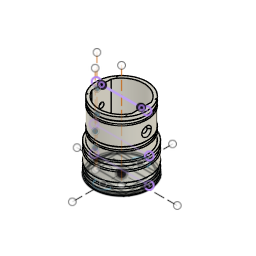
Gehäuse_unten v17 (Autodesk Fusion 360 design; units mm, degrees)
Autodesk Fusion 360 part; units mm, degrees
note: some values were not read from the file. Set by a fixed rule: which sketch regions a step uses; the direction of a hole.
sketch "Skizze1" plane through (0, 0, 0) normal (0, 0, 1) x (1, 0, 0)
  circle A0 centre (0, 0) radius 24.75
  circle A1 centre (0, 0) radius 21.75
  line L0 (-17.5, 13.5) -> (17.5, 13.5)
  line L1 (17.5, 13.5) -> (17.5, -13.5)
  line L2 (17.5, -13.5) -> (-17.5, -13.5)
  line L3 (-17.5, -13.5) -> (-17.5, 13.5)
  line L4 (-40, 0) -> (50, 0) construction
  line L5 (0, 45.7661) -> (0, -44.2339) construction
  line L6 (-18.4476, 16.5) -> (18.4476, 16.5)
  line L7 (20.5, 13.8677) -> (20.5, -13.8677)
  line L8 (18.4476, -16.5) -> (-18.4476, -16.5)
  line L9 (-20.5, -13.8677) -> (-20.5, 13.8677)
  arc A2 (6.5, 16.5) -> (-6.5, 16.5) centre (0, 16.5) ccw
  arc A3 (-6.6213, -16.5) -> (6.3787, -16.5) centre (-0.1213, -16.5) ccw
  arc A4 (-21.6357, 2.2272) -> (-21.6357, -2.2272) centre (-20.5, 0) ccw
  arc A5 (20.5, -2.5) -> (20.5, 2.5) centre (20.5, 0) ccw
  circle A6 centre (0, 0) radius 23 construction
  line L10 (-14.5, -7.5) -> (14.5, -7.5)
  line L11 (14.5, -7.5) -> (14.5, 7.5)
  line L12 (14.5, 7.5) -> (-14.5, 7.5)
  line L13 (-14.5, 7.5) -> (-14.5, -7.5)
  circle A7 centre (0, 0) radius 22.75
  dimension "d1" = 49.5
  dimension "d3" = 3
  dimension "d4" = 27
  dimension "d5" = 35
  dimension "d6" = 3
  dimension "d7" = 3
  dimension "d8" = 3
  dimension "d9" = 3
  dimension "d18" = 46
  dimension "d19" = 29
  dimension "d20" = 15
  dimension "d43" = 45.5
  constraint coincident A0.centre A1.centre
  constraint horizontal L0
  constraint vertical L1
  constraint horizontal L2
  constraint vertical L3
  constraint parallel L2 L4
  constraint symmetric L0 L2 L4
  constraint vertical L5
  constraint symmetric L1 L3 L5
  constraint coincident A0.centre L5
  constraint coincident A0.centre L4
  constraint horizontal L6
  constraint vertical L7
  constraint horizontal L8
  constraint vertical L9
  constraint equal A2 A3
  constraint coincident L6 A2.end
  constraint coincident L6 A2.start
  constraint coincident L8 A3.end
  constraint coincident L8 A3.start
  constraint coincident A0 L8.end
  constraint coincident L8 A3.centre
  constraint coincident A0 L9.start
  constraint coincident A0 L9.end
  constraint coincident A0 L6.start
  constraint coincident L6 A2.centre
  constraint coincident A0 L7.start
  constraint coincident A0 L6.end
  constraint coincident A0 L7.end
  constraint coincident A0 L8.start
  constraint midpoint L9 A4.centre
  constraint midpoint L7 A5.centre
  constraint equal A4 A5
  constraint coincident A1 A4.start
  constraint coincident A1 A4.end
  constraint coincident L7 A5.end
  constraint coincident L7 A5.start
  constraint concentric A0 A6
  constraint tangent A5 A6
  constraint tangent A2 A6
  constraint horizontal L10
  constraint vertical L11
  constraint horizontal L12
  constraint vertical L13
  constraint symmetric L5 L11 L13
  constraint symmetric L4 L10 L12
  constraint concentric A1 A7
  measures "d1" diameter of A0
  measures "d3" distance of A0 A1
  measures "d4" distance of L0.start L2.end
  measures "d5" distance of L0.start L0.end
  measures "d6" distance of L3 L9
  measures "d7" distance of L1 L7
  measures "d8" distance of L0 L6
  measures "d9" distance of L2 L8
  measures "d18" diameter of A6
  measures "d19" distance of L10.start L10.end
  measures "d20" distance of L10.end L11.end
  measures "d43" diameter of A7
extrude "Extrusion1" add sketch "Skizze1" along normal blind 60 contours A0 L7 A5 A7 | A0 L6 L7 A7 | A0 L7 L8 A7 | A0 L6 A2 A7 | A1 L7 A5 A7 | A1 L0 L1 L6 L7 A7 | A0 L8 A3 A7 | A1 L1 L2 L7 L8 A7 | A1 L7 A5 A7 | A0 L6 L9 A7 | A1 L6 A2 A7 | A1 A5 A7 | A5 A7 | A0 L8 L9 A7 | A1 L8 A3 A7 | A0 L9 A4 A7 | A1 L6 A2 A7 | A1 L0 L3 L6 L9 A7 | A2 A7 | A1 A2 A7 | A1 L2 L3 L8 L9 A7 | A1 L8 A3 A7 | A1 A3 A7 | A3 A7 | A1 L9 A4 A7 | A1 L9 A4 A7 | A4 A7 | A1 A4 A7
extrude "Extrusion2" add sketch "Skizze1" along normal blind 3 contours A1 L1 L7 | A1 L7 A5 | A1 L7 A5 | A1 L6 A2 | A1 L0 L6 | A1 L7 A5 | A1 L0 L1 L2 L3 | A1 L2 L8 | A1 L8 A3 | A1 L6 A2 | A1 L6 A2 | A1 L8 A3 | A1 L8 A3 | A1 L9 | A1 L3 L9 | L10 L11 L12 L13
chamfer "Fase1" distance 3 angle 12 1 edges at (-23.0751, -8.95, 0) measured on face at (24.627, -2.4643, 20)
extrude "Extrusion3" cut sketch "Skizze1" along normal up to surface (3 mm away) contours L10 L11 L12 L13
extrude "Extrusion4" add sketch "Skizze1" along normal up to surface (60 mm away) contours A1 L7 A5 | A1 L7 A5 | A1 L7 A5 | A1 L9
chamfer "Fase2" distance 1.5 angle 45 4 edges at (0, -7.5, 3) (-14.5, 0, 3) (0, 7.5, 3) (14.5, 0, 3) measured on face at (-0.5022, -12.2326, 3) measured on face at (-0.5022, -12.2326, 3) measured on face at (-0.5022, -12.2326, 3) measured on face at (-0.5022, -12.2326, 3)
sketch "Skizze2" plane through (-20.5, 0, 0) normal (1, 0, 0) x (0, 1, 0)
  line L0 (-7.2672, 3) -> (7.2672, 3)
  line L1 (7.2672, 3) -> (7.2672, 60)
  line L2 (7.2672, 60) -> (-7.2672, 60)
  line L3 (-7.2672, 60) -> (-7.2672, 3)
  line L4 (7.2672, 3) -> (12.9156, 3)
  line L5 (13.5, 3) -> (12.9156, 3)
  line L6 (13.5, 3) -> (21.75, 3)
  line L7 (13.5, 3) -> (12.9156, 3)
  line L8 (7.2672, 3) -> (12.9156, 3)
  line L9 (7.2672, 3) -> (-7.2672, 3)
  line L10 (-12.9156, 3) -> (-7.2672, 3)
  line L11 (-12.9156, 3) -> (-13.5, 3)
  line L12 (-21.75, 3) -> (-13.5, 3)
  line L13 (-12.9156, 3) -> (-13.5, 3)
  line L14 (-12.9156, 3) -> (-7.2672, 3)
  line L15 (-7.2672, 3) -> (7.2672, 3)
  line L16 (-9, 3) -> (9, 3)
  line L17 (9, 3) -> (-9, 3)
  line L18 (-21.75, 60) -> (-13.5, 60)
  line L19 (-13.5, 60) -> (-12.9156, 60)
  line L20 (-12.9156, 60) -> (-7.2672, 60)
  line L21 (-7.2672, 60) -> (7.2672, 60)
  line L22 (7.2672, 60) -> (12.9156, 60)
  line L23 (12.9156, 60) -> (13.5, 60)
  line L24 (13.5, 60) -> (21.75, 60)
  line L25 (13.5, 60) -> (12.9156, 60)
  line L26 (7.2672, 60) -> (12.9156, 60)
  line L27 (7.2672, 60) -> (-7.2672, 60)
  line L28 (-12.9156, 60) -> (-7.2672, 60)
  line L29 (-12.9156, 60) -> (-13.5, 60)
  line L30 (24.75, 60) -> (-24.75, 60)
  circle A0 centre (0, 44) radius 2.25
  line L31 (0, 60) -> (0, 3) construction
  dimension "d30" = 4.5
  dimension "d31" = 41
  constraint midpoint L21 L31.start
  constraint coincident A0.centre L31
  measures "d30" diameter of A0
  measures "d31" distance of L0 A0.centre
extrude "Extrusion5" cut sketch "Skizze2" along normal blind 110 and the other way blind 40 contours A0
hole "Bohrung1" at (-0.1213, -16.5, 0) at (20.5, 0, 0) at (0, 16.5, 0) at (-20.5, 0, 0) direction (0, 0, 1) diameter 2 depth 8 tip angle 118
sketch "Skizze4" plane through (0, 0, 3) normal (0, 0, 1) x (-1, 0, 0)
  arc A0 (-20.5, -1) -> (-20.5, 1) centre (-20.5, 0) ccw
  line L0 (-20.5, -1) -> (-20.5, -7.2672)
  arc A1 (-20.5, -7.2672) -> (-17.5, -12.9156) centre (0, 0) ccw
  arc A2 (-17.5, -12.9156) -> (-17.0532, -13.5) centre (0, 0) ccw
  arc A3 (-17.0532, -13.5) -> (17.0532, -13.5) centre (0, 0) ccw
  arc A4 (17.0532, -13.5) -> (17.5, -12.9156) centre (0, 0) ccw
  arc A5 (17.5, -12.9156) -> (20.5, -7.2672) centre (0, 0) ccw
  line L1 (20.5, -7.2672) -> (20.5, -1)
  arc A6 (20.5, 1) -> (20.5, -1) centre (20.5, 0) ccw
  line L2 (20.5, 1) -> (20.5, 7.2672)
  arc A7 (20.5, 7.2672) -> (17.5, 12.9156) centre (0, 0) ccw
  arc A8 (17.5, 12.9156) -> (17.0532, 13.5) centre (0, 0) ccw
  arc A9 (17.0532, 13.5) -> (-17.0532, 13.5) centre (0, 0) ccw
  arc A10 (-17.0532, 13.5) -> (-17.5, 12.9156) centre (0, 0) ccw
  arc A11 (-17.5, 12.9156) -> (-20.5, 7.2672) centre (0, 0) ccw
  line L3 (-20.5, 7.2672) -> (-20.5, 1)
  circle A12 centre (0, -16.5) radius 1
  circle A13 centre (0.1213, 16.5) radius 1
  line L4 (-16, 9) -> (16, 9)
  line L5 (16, 9) -> (16, -9)
  line L6 (16, -9) -> (-16, -9)
  line L7 (-16, -9) -> (-16, 9)
  line L8 (20.5, -2.25) -> (20.5, 2.25)
  line L9 (20.5, 1) -> (20.5, 0)
  line L10 (20.5, 0) -> (20.5, -1)
  line L11 (20.5, -1) -> (20.5, -7.2672)
  line L12 (20.5, -7.2672) -> (20.5, 7.2672)
  line L13 (20.5, 7.2672) -> (20.5, 1)
  arc A14 (17.5, -12.9156) -> (20.5, -7.2672) centre (0, 0) ccw
  arc A15 (17.5, -12.9156) -> (20.5, -7.2672) centre (0, 0) ccw
  arc A16 (-17.0532, -13.5) -> (17.0532, -13.5) centre (0, 0) ccw
  arc A17 (-17.0532, -13.5) -> (17.0532, -13.5) centre (0, 0) ccw
  arc A18 (20.5, 7.2672) -> (17.5, 12.9156) centre (0, 0) ccw
  arc A19 (20.5, 7.2672) -> (17.5, 12.9156) centre (0, 0) ccw
  arc A20 (-20.5, -7.2672) -> (-17.5, -12.9156) centre (0, 0) ccw
  arc A21 (-20.5, -7.2672) -> (-17.5, -12.9156) centre (0, 0) ccw
  line L14 (-20.5, 2.25) -> (-20.5, -2.25)
  line L15 (-20.5, -1) -> (-20.5, 0)
  line L16 (-20.5, 0) -> (-20.5, 1)
  line L17 (-20.5, 1) -> (-20.5, 7.2672)
  line L18 (-20.5, 7.2672) -> (-20.5, -7.2672)
  line L19 (-20.5, -7.2672) -> (-20.5, -1)
  arc A22 (-17.5, 12.9156) -> (-20.5, 7.2672) centre (0, 0) ccw
  arc A23 (-17.5, 12.9156) -> (-20.5, 7.2672) centre (0, 0) ccw
  arc A24 (17.0532, 13.5) -> (-17.0532, 13.5) centre (0, 0) ccw
  arc A25 (17.0532, 13.5) -> (-17.0532, 13.5) centre (0, 0) ccw
  circle A26 centre (0, -16.5) radius 1
  circle A27 centre (0.1213, 16.5) radius 1
  circle A28 centre (0, 0) radius 20
  line L20 (18, -8.7178) -> (18, 8.7178)
  line L21 (-18, -8.7178) -> (-18, 8.7178)
  point P0 (20.5, -21.75)
  dimension "d47" = 40
  dimension "d48" = 36
  constraint concentric A20 A28
  constraint coincident A28 L20.start
  constraint coincident A28 L20.end
  constraint vertical L20
  constraint coincident A28 L21.start
  constraint coincident A28 L21.end
  constraint vertical L21
  constraint equal L20 L21
  measures "d47" diameter of A28
  measures "d48" distance of L20 L21
extrude "Extrusion7" add sketch "Skizze4" along normal up to surface (57 mm away) contours A0 L14 L15 L16 L18 A28 | A0 L0 A1 A2 A3 A4 A5 L1 A6 L8 L11 L12 A14 A15 A16 A17 A20 A21 L14 L18 L19 A28 | A0 A28 | A0 A28 L21 | A0 A6 L2 A7 A8 A9 A10 A11 L3 L8 L12 L13 A18 A19 L14 L17 L18 A22 A23 A24 A25 A28 | A6 A28 L20 | A6 L8 L9 L10 L12 A28 | A6 A28
extrude "Extrusion6" cut sketch "Skizze1" along normal up to surface (34 mm away) from surface at 26 contours A0 L7 A5 A7 | A0 L6 L7 A7 | A0 L7 L8 A7 | A0 L6 A2 A7 | A0 L8 A3 A7 | A0 L6 L9 A7 | A5 A7 | A0 L8 L9 A7 | A0 L9 A4 A7 | A2 A7 | A3 A7 | A4 A7
extrude "Extrusion8" cut sketch "Skizze2" along normal blind 55 contours A0
sketch "Skizze3" plane through (0, 0, 0) normal (0, 1, 0) x (1, 0, 0)
  line L0 (-17.0532, -60) -> (-17.5, -60)
  line L1 (-17.5, -60) -> (-17.0532, -60)
  line L2 (17.0532, -60) -> (17.5, -60)
  line L3 (17.5, -60) -> (17.0532, -60)
  line L4 (-22.1, -83.0309) -> (-22.1, 7) construction
  line L5 (0, -84) -> (0, 9) construction
  circle A0 centre (-22.1, -55) radius 1.1
  circle A1 centre (-22.1, -35) radius 1.1
  line L6 (-22.75, -60) -> (22.75, -60)
  line L7 (17.5, -60) -> (17.0532, -60)
  line L8 (17.5, -60) -> (17.0532, -60)
  line L9 (-17.0532, -60) -> (-17.5, -60)
  line L10 (-18, -60) -> (18, -60)
  line L11 (-18, -60) -> (18, -60)
  line L12 (-17.0532, -60) -> (-17.5, -60)
  circle A2 centre (-23.7, -21) radius 1.6
  circle A3 centre (-23.7, -8) radius 1.6
  line L13 (-23.7, 9.1317) -> (-23.7, -70) construction
  line L14 (24.75, -3) -> (-24.75, -3)
  line L15 (24.75, -26) -> (-24.75, -26)
  dimension "d38" = 22.1
  dimension "d39" = 2.2
  dimension "d56" = 3.2
  dimension "d57" = 5
  dimension "d58" = 5
  dimension "d59" = 23.7
  constraint vertical L5
  constraint coincident L4 A0.centre
  constraint coincident L4 A1.centre
  constraint equal A0 A1
  constraint vertical L13
  constraint coincident A3.centre L13
  constraint coincident A2.centre L13
  constraint equal A2 A3
  measures "d38" distance of L4 L5
  measures "d39" diameter of A0
  measures "d56" diameter of A2
  measures "d57" distance of A3.centre L14
  measures "d58" distance of A2.centre L15
  measures "d59" distance of L5 L13
revolve "Drehen2" cut sketch "Skizze3" angle 360 about axis through (0, 0, 84) along (0, 0, -1) contours A0 | A1
revolve "Drehen3" cut sketch "Skizze3" angle 360 about axis through (0, 0, 84) along (0, 0, -1) contours A2 | A3
fillet "Abrundung1" radius 0.75 8 edges at (-21.2104, -8.2268, 55.8874) (-21.2104, 8.2268, 54.1126) (-21.2104, -8.2268, 35.8874) (-21.2104, 8.2268, 34.1126) (-23.0751, -8.95, 22.2073) (-23.0751, 8.95, 19.7927) (-23.0751, -8.95, 9.2073) (-23.0751, 8.95, 6.7927)
chamfer "Fase4" distance 2 angle 45 2 edges at (-22.6385, -2.25, 44) (22.6385, -2.25, 44)
equation "d38 = ( 45.5 / 2 ) * 1 mm - 0.65 mm"
equation "d59 = ( 49 / 2 ) * 1 mm - 0.8 mm"
